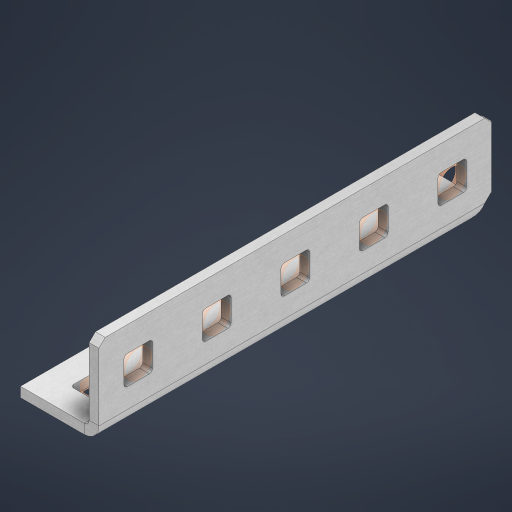
# Autodesk Inventor part: Alu C 1x3x1x35
Saved by Autodesk Inventor 2023 (Build 270158000, 158)
## iProperties
Created: 2022-07-28
Part Number: Alu C 1x3x1x35
Material: Generic
Document SubType Name: Sheet Metal
Designer: ylu12
Density: 1 g/cm^3
Sheet Metal Rule: Default
Appearance: Alu
Author: ylu12
Autodesk Inventor part; units mm, degrees
ref_plane "YZ Plane" through (0, 0, 0) normal (1, 0, 0) x (0, 1, 0)
ref_plane "XZ Plane" through (0, 0, 0) normal (0, 1, 0) x (-1, 0, 0)
ref_plane "XY Plane" through (0, 0, 0) normal (0, 0, 1) x (1, 0, 0)
sketch "Sketch1" plane through (0, 0, 0) normal (0, 1, 0) x (-1, 0, 0)
  line L0 (-19.05, 0) -> (19.05, 0)
  line L1 (19.05, 0) -> (19.05, -63.5)
  line L2 (19.05, -63.5) -> (-19.05, -63.5)
  line L3 (-19.05, -63.5) -> (-19.05, 0)
  line L4 (19.05, 0) -> (-19.05, -63.5) construction
  point P0 (0, 0)
  point P1 (0, 0)
  dimension "d0" = 38.1
  dimension "d1" = 63.5
  measures "d0" distance of L1.end L2.end
  measures "d1" distance of L0.end L1.end
extrude "Plate1" add sketch "Sketch1" along normal blind 1.5875
sketch "Sketch2" plane through (17.4625, 0, -63.5) normal (1, 0, 0) x (0, 1, 0)
  line L0 (0, 63.5) -> (0, 0)
  line L1 (0, 0) -> (14.2875, 0)
  line L2 (14.2875, 0) -> (14.2875, 63.5)
  line L3 (14.2875, 63.5) -> (0, 63.5)
  constraints: 6 end point, 1 horizontal, 1 perpendicular, 1 vertical
edge flange "Flanges" height 12.7 angle 90 thickness 1.5875 bend radius 0.7937 thickness toward (1, 0, 0) relief straight relief width 1.5875 relief depth 0.7937 corner gap 1.5875 corner form 0 edges at (19.05, 1.5875, -31.75) (-19.05, 1.5875, -31.75) wall of the first edge with corners at (17.4625, 0, 0) (17.4625, 0, -63.5) (17.4625, 14.2875, -63.5) (17.4625, 14.2875, 0)
bend "Bend1"
corner "Corner1"
sketch "Sketch3" plane through (19.05, 2.3813, -63.5) normal (1, 0, 0) x (0, 0, -1)
  line L0 (-58.9534, 7.8676) -> (-55.3466, 7.8676)
  line L1 (-54.8386, 7.3596) -> (-54.8386, 3.7529)
  line L2 (-55.3466, 3.2449) -> (-58.9534, 3.2449)
  line L3 (-59.4614, 3.7529) -> (-59.4614, 7.3596)
  arc A0 (-58.9534, 7.8676) -> (-59.4614, 7.3596) centre (-58.9534, 7.3596) ccw
  arc A1 (-54.8386, 7.3596) -> (-55.3466, 7.8676) centre (-55.3466, 7.3596) ccw
  arc A2 (-55.3466, 3.2449) -> (-54.8386, 3.7529) centre (-55.3466, 3.7529) ccw
  arc A3 (-59.4614, 3.7529) -> (-58.9534, 3.2449) centre (-58.9534, 3.7529) ccw
  line L4 (-63.5, 0) -> (-63.5, 11.9062) construction
  line L5 (-63.5, 11.9062) -> (0, 11.9062) construction
  line L6 (-58.9534, 7.3596) -> (-55.3466, 3.7529) construction
  point P0 (-63.5, -2.3813)
  point P1 (-54.8386, 3.2449)
  point P2 (-59.4614, 3.2449)
  point P3 (-57.15, 5.5563)
  dimension "d16" = 4.6228
  dimension "d17" = 0.508
  dimension "d20" = 6.35
  dimension "d21" = 6.35
  constraints: 10 end point, 8 point on circle, 8 tangent, 4 centre point, 4 point on line, 3 equal radius, 2 parallel, 2 perpendicular, 1 horizontal, 1 midpoint
  measures "d16" distance of point (-54.839, 3.245) point (-59.461, 3.245)
  measures "d17" radius of A0
  measures "d20" distance from line of point (-57.15, 5.556) L4
  measures "d21" distance from line of L5 point (-57.15, 5.556)
extrude "Flange Stamp" cut sketch "Sketch3" against normal blind 1.5875
sketch "Sketch7" plane through (19.05, 2.3813, 0) normal (1, 0, 0) x (0, 0, -1)
  arc A0 (4.5466, 7.8676) -> (4.0386, 7.3596) centre (4.5466, 7.3596) ccw construction
  arc A1 (8.1534, 3.2449) -> (8.6614, 3.7529) centre (8.1534, 3.7529) ccw construction
  circle A2 centre (6.35, 5.5563) radius 2.1844
  line L0 (4.5466, 7.3596) -> (8.1534, 3.7529) construction
  point P0 (0, -2.3813)
  dimension "d46" = 4.3688
  constraints: 2 end point, 1 centre point, 1 midpoint
  measures "d46" diameter of A2
surface extrude "Flange Circle" sketch "Sketch7" against normal up to surface (1.5875 mm away) shown yes curves A2
ref_plane "Flange Pattern Plane" through (19.05, 7.9375, -4.5466) normal (0, 1, 0) x (1, 0, 0)
sketch "Flange Pattern Sketch" plane through (19.05, 7.9375, -4.5466) normal (0, 1, 0) x (1, 0, 0)
  line L0 (0, 3.6068) -> (0, 0) construction
  line L1 (-45.8186, -4.5466) -> (8.2118, -4.5466) construction
  line L2 (0, 0) -> (-1.5875, 0) construction
  point P0 (-19.05, -4.5466)
  point P1 (0, 1.8034)
  point P2 (0, 14.5034)
  point P3 (0, 27.2034)
  point P4 (0, 39.9034)
  point P5 (0, 52.6034)
  dimension "d131" = 12.7
  dimension "d134" = 12.7
  constraints: 1 horizontal, 1 midpoint, 1 vertical, 4 other
  measures "d134" distance of point (0, 1.803) point (0, 14.503)
pattern_sketch "Flange Pattern" of "Flange Circle", "Flange Stamp" from (19.05, 7.9375, -6.35) copies at (19.05, 7.9375, -19.05) at (19.05, 7.9375, -31.75) at (19.05, 7.9375, -44.45) at (19.05, 7.9375, -57.15)
sketch "Sketch8" plane through (0, 0, 0) normal (0, -1, 0) x (1, 0, 0)
  line L0 (16.6687, 0) -> (-16.6687, 0) construction
  line L1 (14.5034, -4.0386) -> (10.8966, -4.0386)
  line L2 (10.3886, -4.5466) -> (10.3886, -8.1534)
  line L3 (10.8966, -8.6614) -> (14.5034, -8.6614)
  line L4 (15.0114, -8.1534) -> (15.0114, -4.5466)
  arc A0 (15.0114, -4.5466) -> (14.5034, -4.0386) centre (14.5034, -4.5466) ccw
  arc A1 (14.5034, -8.6614) -> (15.0114, -8.1534) centre (14.5034, -8.1534) ccw
  arc A2 (10.3886, -8.1534) -> (10.8966, -8.6614) centre (10.8966, -8.1534) ccw
  arc A3 (10.8966, -4.0386) -> (10.3886, -4.5466) centre (10.8966, -4.5466) ccw
  line L5 (14.5034, -4.5466) -> (10.8966, -8.1534) construction
  line L6 (19.05, 0) -> (19.05, -63.5) construction
  point P0 (0, 0)
  point P1 (10.3886, -8.6614)
  point P2 (15.0114, -8.6614)
  point P3 (12.7, -6.35)
  dimension "d49" = 4.6228
  dimension "d50" = 0.508
  dimension "d51" = 6.35
  dimension "d52" = 6.35
  constraints: 10 end point, 8 point on circle, 8 tangent, 4 centre point, 4 point on line, 3 equal radius, 2 parallel, 2 perpendicular, 1 horizontal, 1 midpoint
  measures "d49" distance of point (15.011, -8.661) point (10.389, -8.661)
  measures "d50" radius of A0
  measures "d51" distance from line of L6 point (12.7, -6.35)
  measures "d52" distance from line of L0 point (12.7, -6.35)
extrude "Body Stamp" cut sketch "Sketch8" against normal blind 1.5875
sketch "Sketch9" plane through (0, 0, 0) normal (0, -1, 0) x (1, 0, 0)
  arc A0 (15.0114, -4.5466) -> (14.5034, -4.0386) centre (14.5034, -4.5466) ccw construction
  arc A1 (10.3886, -8.1534) -> (10.8966, -8.6614) centre (10.8966, -8.1534) ccw construction
  line L0 (14.5034, -4.5466) -> (10.8966, -8.1534) construction
  circle A2 centre (12.7, -6.35) radius 2.1844
  point P0 (0, 0)
  dimension "d55" = 4.3688
  constraints: 2 end point, 1 centre point, 1 midpoint
  measures "d55" diameter of A2
surface extrude "Body Circle" sketch "Sketch9" against normal up to surface (1.5875 mm away) shown yes curves A2
sketch "Body Pattern Sketch" plane through (0, 0, 0) normal (0, -1, 0) x (1, 0, 0)
  line L0 (16.6687, 0) -> (-16.6687, 0) construction
  line L1 (19.05, 0) -> (19.05, -63.5) construction
  circle A0 centre (12.7, -6.35) radius 2.1844 construction
  point P0 (0, 0)
  point P1 (12.7, -19.05)
  point P2 (12.7, -31.75)
  point P3 (12.7, -44.45)
  point P4 (12.7, -57.15)
  dimension "d62" = 12.7
  dimension "d65" = 12.7
  dimension "d139" = 12.7
  constraints: 1 coincident, 1 horizontal, 1 vertical, 4 other
  measures "d139" distance of point (12.7, -19.05) point (12.7, -6.35)
pattern_sketch "Body Pattern" of "Body Stamp", "Body Circle" from (12.7, 0, -6.35) copies at (12.7, 0, -19.05) at (12.7, 0, -31.75) at (12.7, 0, -44.45) at (12.7, 0, -57.15)
sketch "Arc Length" plane through (17.4625, 2.3812, 0) normal (0, 0, 1) x (1, 0, 0)
  line L0 (0, 0) -> (1.5875, 0) construction
  arc A0 (-0.7937, -0.7937) -> (0, 0) centre (-0.7937, 0) ccw construction
  line L1 (-0.7938, -2.3812) -> (-0.7937, -0.7937) construction
  arc A1 (-0.7938, -2.3812) -> (1.5875, 0) centre (-0.7937, 0) ccw construction
  point P0 (-17.4625, -2.3812)
  dimension "d85" = 3.7405
  dimension "d92" = 1.2468
sketch "Sketch13" plane through (19.05, 14.2875, 0) normal (1, 0, 0) x (0, 0, -1)
  line L0 (0, 0) -> (63.5, 0) construction
  line L1 (62.4078, 0) -> (63.4238, -1.016)
  line L2 (63.4238, -1.016) -> (64.4398, 0)
  line L3 (62.4078, 0) -> (64.4398, 0)
  line L4 (63.5, -11.9062) -> (0, -11.9062) construction
  line L5 (63.4238, -10.8903) -> (61.161, -13.1531)
  line L6 (61.161, -13.1531) -> (63.4238, -15.4159)
  line L7 (63.4238, -15.4159) -> (65.6866, -13.1531)
  line L8 (65.6866, -13.1531) -> (63.4238, -10.8903)
  line L9 (63.4238, -10.8903) -> (63.4238, -15.4159) construction
  line L10 (63.4238, -1.016) -> (63.4238, -10.8903) construction
  line L11 (0, -11.9062) -> (63.5, -11.9062) construction
  point P0 (0, -14.2875)
  dimension "d86" = 4.5256
  dimension "d88" = 1.016
  dimension "d91" = 1.016
  dimension "d102" = 63.4238
  constraints: 19 end point, 6 perpendicular, 2 point on line, 2 vertical, 1 collinear
  measures "d86" distance of L5.start L6.end
  measures "d88" distance from line of L0 L1.end
  measures "d91" distance from line of L5.start L11
  measures "d102" distance from line of L0.start L10
cut across bends "Notch" sketch "Sketch13" k factor 0.44
mirror "Notch Mirror" [suppressed]
pattern_linear "Notch Pattern" [suppressed]
chamfer "End Chamfer" distance 1.016 angle 45 3 edges at (-18.2562, 14.2875, 0) (18.2562, 14.2875, 0) (-18.2562, 14.2875, -63.5)
sketch "Sketch14" plane through (-19.05, 2.3813, 381) normal (1, 0, 0) x (0, 0, -1)
  line L0 (381, 11.9063) -> (444.5, 11.9063) construction
  line L1 (381, 0) -> (381, 11.9063) construction
  line L2 (381, -2.3813) -> (444.5, -2.3813) construction
  line L3 (381, 11.9063) -> (444.5, 11.9063)
  line L4 (444.5, 11.9063) -> (444.5, -2.3813)
  line L5 (444.5, -2.3813) -> (381, -2.3813)
  line L6 (381, -2.3813) -> (381, 11.9063)
  point P0 (381, -2.3812)
  point P1 (382.0521, -1.9844)
  constraints: 8 end point, 2 collinear, 2 parallel, 1 horizontal, 1 perpendicular, 1 other
extrude "Half Cut" cut sketch "Sketch14" along normal blind 25.4
equation "\"d1\" = 12.7 * Length"
equation "\"d18\" = Thickness"
equation "\"d53\" = Thickness"
equation "\"d89\" = Thickness"
equation "\"d2\" = Thickness"
equation "\"d3\" = BendReliefWidth"
equation "\"d4\" = BendReliefDepth"
equation "\"d5\" = MinimumRemnant"
equation "\"d6\" = TransitionRadius"
equation "\"d10\" = CornerReliefSize"
equation "\"d11\" = GapSize"
equation "\"d12\" = JacobiRadiusSize"
equation "\"BendRadius\" = Thickness"
equation "\"BendReliefWidth\" = Thickness"
equation "\"BendReliefDepth\" = 0.5 * Thickness"
equation "\"CornerReliefSize\" = 4 * Thickness"
equation "\"MinimumRemnant\" = 2 * Thickness"
equation "\"TransitionRadius\" = BendRadius"
equation "\"JacobiRadiusSize\" = BendRadius"
equation "\"GapSize\" = Thickness"
equation "\"Length\" = 5"
equation "\"Thickness\" = 1.5875"
body "Solid1"
body "Srf1"
body "Srf2"
body "Srf91"
body "Srf92"
body "Srf856"
body "Srf1310"
body "Srf1311"
body "Srf1312"
body "Srf1376"
body "Srf1377"
